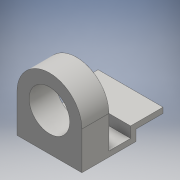
# Autodesk Inventor part: ProbeMount
Saved by Autodesk Inventor 2016 (Build 200138000, 138)
## iProperties
Created: 2015-11-05
Part Number: ProbeMount
Material: Generic
Document SubType Name: Modeling
Designer: PowerStation9000
Density: 1 g/cm^3
Appearance: Default
Author: PowerStation9000
Autodesk Inventor part; units mm, degrees
ref_plane "YZ Plane" through (0, 0, 0) normal (1, 0, 0) x (0, 1, 0)
ref_plane "XZ Plane" through (0, 0, 0) normal (0, 1, 0) x (-1, 0, 0)
ref_plane "XY Plane" through (0, 0, 0) normal (0, 0, 1) x (1, 0, 0)
sketch "Sketch1" plane through (0, 0, 0) normal (0, 0, 1) x (1, 0, 0)
  line L0 (-12, 5) -> (12, 5)
  line L1 (12, 5) -> (12, -5)
  line L2 (12, -5) -> (-12, -5)
  line L3 (-12, -5) -> (-12, 5)
  point P0 (0, 0)
  dimension "d0" = 24
  dimension "d1" = 10
  dimension "d2" = 5
  dimension "d3" = 12
  constraints: 8 end point, 2 parallel, 1 horizontal, 1 perpendicular
  measures "d0" distance of L1.end L2.end
  measures "d1" distance of L0.end L1.end
  measures "d2" distance from line of point (0, 0) L0
  measures "d3" distance from line of point (0, 0) L1
extrude "Extrusion1" add sketch "Sketch1" along normal blind 28
sketch "Sketch2" plane through (-12, 5, 0) normal (0, 1, 0) x (1, 0, 0)
  line L0 (0, 0) -> (24, 0) projected
  line L1 (0, 0) -> (0, -28) projected
  line L2 (24, -28) -> (0, -28) projected
  line L3 (24, 0) -> (24, -28) projected
  circle A0 centre (12, -14) radius 7.5
  point P0 (12, 0)
  dimension "d6" = 15
  dimension "d7" = 28
  dimension "d8" = 24
  dimension "d9" = 12
  dimension "d10" = 14
  constraints: 1 centre point
  measures "d6" diameter of A0
  measures "d7" distance of L0.start L1.end
  measures "d8" distance of L0.start L0.end
  measures "d9" distance from line of L1 A0.centre
  measures "d10" distance from line of L0 A0.centre
extrude "Extrusion2" cut sketch "Sketch2" against normal up to next contours A0
sketch "Sketch7" plane through (-12, 5, 28) normal (0, 1, 0) x (1, 0, 0)
  circle A0 centre (12, 14) radius 7.5 projected
  line L0 (0, 28) -> (0, 0) projected
  line L1 (24, 0) -> (0, 0) projected
  line L2 (24, 28) -> (24, 0) projected
  arc A1 (0, 14) -> (24, 14) centre (12, 14) ccw
  line L3 (24, 32) -> (24, 0) projected
  line L4 (24, 32) -> (24, 0) projected
  line L5 (24, 14) -> (24, 0)
  line L6 (24, 0) -> (0, 0)
  line L7 (24, 0) -> (0, 0) projected
  line L8 (0, 0) -> (0, 14)
  line L9 (0, 32) -> (0, 0) projected
  line L10 (0, 28) -> (24, 28) projected
  point P0 (12, 28)
  constraints: 6 end point, 4 tangent, 2 point on circle, 2 point on line, 1 centre point, 1 coincident, 1 collinear, 1 perpendicular
extrude "Extrusion6" cut sketch "Sketch7" against normal blind 20 contours A1 L2 L1 L0
sketch "Sketch9" plane through (-12, -5, 0) normal (-1, 0, 0) x (0, 0, 1)
  line L0 (14, 0) -> (14, 10) construction
  line L1 (0, 10) -> (14, 10) construction
  line L2 (0, 0) -> (0, 10) construction
  line L3 (0, 0) -> (14, 0) construction
  line L4 (0, 10) -> (14, 10) projected
  line L5 (0, 10) -> (0, 20)
  line L6 (0, 20) -> (4, 20)
  line L7 (4, 20) -> (4, 30)
  line L8 (4, 30) -> (6, 30)
  line L9 (6, 30) -> (6, 18)
  line L10 (6, 18) -> (2, 18)
  line L11 (2, 18) -> (2, 10)
  line L12 (0, 10) -> (2, 10)
  point P0 (0, 5)
  dimension "d32" = 10
  dimension "d33" = 4
  dimension "d34" = 10
  dimension "d35" = 2
  dimension "d36" = 2
  dimension "d37" = 2
  constraints: 16 end point, 7 perpendicular, 1 point on line, 1 vertical
  measures "d32" distance of L1.start L5.end
  measures "d33" distance of L5.end L6.end
  measures "d34" distance of L6.end L7.end
  measures "d35" distance between parallel lines of L7 L9
  measures "d36" distance between parallel lines of L6 L10
  measures "d37" distance between parallel lines of L5 L11
extrude "Extrusion8" add sketch "Sketch9" against normal up to surface (24 mm away)
equation "\"d2\" = 0.5 * d1"
equation "\"d3\" = 0.5 * d0"
equation "\"d9\" = 0.5 * d8"
equation "\"d10\" = 0.5 * d7"
body "Solid1"
